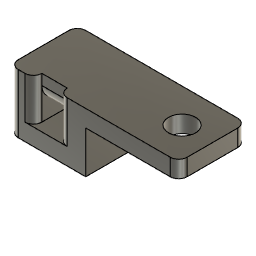
b_tail_mount (Autodesk Fusion 360 design; units mm, degrees)
Autodesk Fusion 360 part; units mm, degrees
sketch "Sketch1" plane through (0, 0, 0) normal (0, 0, 1) x (1, 0, 0)
  line L0 (0, 0) -> (7.4, 0) construction
  circle A0 centre (7.4, 0) radius 1.6
  line L1 (9, -4) -> (-9, -4)
  line L2 (-9, -4) -> (-9, 4)
  line L3 (-9, 4) -> (9, 4)
  line L4 (9, -4) -> (-9, 4) construction
  line L5 (-9, -4) -> (9, 4) construction
  line L6 (9, -4) -> (11, -4)
  line L7 (11, -4) -> (11, 4)
  line L8 (11, 4) -> (9, 4)
  line L9 (0, -4) -> (0, 4)
  dimension "d1" = 7.4
  dimension "d2" = 3.2
  dimension "d3" = 8
  dimension "d4" = 2
  constraint coincident L0.start origin
  constraint horizontal L0
  constraint coincident L0.end A0.centre
  constraint horizontal L1
  constraint perpendicular L1 L2
  constraint parallel L1 L3
  constraint coincident L4 L0.start
  constraint coincident L5 L0.start
  constraint horizontal L6
  constraint vertical L7
  constraint horizontal L8
  constraint midpoint L1 L9.start
  constraint midpoint L3 L9.end
  constraint perpendicular L3 L9
  measures "d1" distance of L0.start L0.end
  measures "d2" diameter of A0
  measures "d3" distance of L1.end L2.end
  measures "d4" distance of L1.start L6.end
extrude "Extrude1" add sketch "Sketch1" along normal blind 2
extrude "Extrude2" add sketch "Sketch1" against normal blind 5 contours L1 L2 L3 L9
fillet "Fillet1" radius 1 4 edges at (11, -4, 1) (11, 4, 1) (-9, -4, -1.5) (-9, 4, -1.5)
sketch "Sketch2" plane through (0, -4, 0) normal (0, -1, 0) x (1, 0, 0)
  line L0 (-8, 2) -> (-8, -5)
  line L1 (-8, -5) -> (0, -5)
  line L2 (0, -5) -> (0, 0)
  line L3 (0, 0) -> (10, 0)
  line L4 (10, 0) -> (10, 2)
  line L5 (10, 2) -> (-8, 2)
  line L6 (-6.2, -1) -> (-3.2, -1)
  line L7 (-3.2, -1) -> (-3.2, -3)
  line L8 (-3.2, -3) -> (-6.2, -3)
  line L9 (-6.2, -3) -> (-6.2, -1)
  dimension "d11" = 3
  dimension "d12" = 2
  constraint horizontal L6
  constraint vertical L7
  constraint horizontal L8
  constraint vertical L9
  measures "d11" distance of L6.start L6.end
  measures "d12" distance of L6.start L8.end
extrude "Extrude3" cut sketch "Sketch2" against normal blind 8 contours L6 L7 L8 L9
sketch "Sketch3" plane through (0, -4, 0) normal (0, -1, 0) x (1, 0, 0)
  line L0 (-3.2, -1) -> (-3.2, -3)
  line L1 (-3.2, -3) -> (-6.2, -3)
  line L2 (-6.2, -3) -> (-6.2, -1)
  line L3 (-6.2, -1) -> (-3.2, -1)
  line L4 (-8, 2) -> (-8, -5)
  line L5 (-8, -5) -> (0, -5)
  line L6 (0, -5) -> (0, 0)
  line L7 (0, 0) -> (10, 0)
  line L8 (10, 0) -> (10, 2)
  line L9 (10, 2) -> (-8, 2)
  line L10 (-6.2, -1) -> (-3.2, -1)
  line L11 (-3.2, -1) -> (-3.2, 2)
  line L12 (-3.2, 2) -> (-6.2, 2)
  line L13 (-6.2, 2) -> (-6.2, -1)
  constraint horizontal L10
  constraint vertical L11
  constraint horizontal L12
  constraint vertical L13
  constraint coincident L9 L11.end
  constraint coincident L2.end L3.start
extrude "Extrude4" cut sketch "Sketch3" against normal blind 1 contours L3 L9 L10 L11 L12 L13
fillet "Fillet3" radius 1 2 edges at (-6.2, -4, -0.5) (-3.2, -4, -0.5)
fillet "Fillet4" radius 1.75 2 edges at (-4.7, -3, -1) (-4.7, 4, -1)
fillet "Fillet2" [suppressed]
